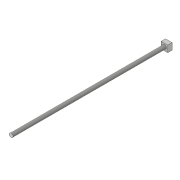
# Autodesk Inventor part: SA
Saved by Autodesk Inventor 2019 (Build 230136000, 136)
## iProperties
Created: 2019-10-07
Part Number: SA
Material: Generic
Document SubType Name: Modeling
Designer: Admin
Density: 1 g/cm^3
Appearance: Default
Author: Admin
Autodesk Inventor part; units mm, degrees
ref_plane "YZ Plane" through (0, 0, 0) normal (1, 0, 0) x (0, 1, 0)
ref_plane "XZ Plane" through (0, 0, 0) normal (0, 1, 0) x (-1, 0, 0)
ref_plane "XY Plane" through (0, 0, 0) normal (0, 0, 1) x (1, 0, 0)
sketch "Sketch1" plane through (0, 0, 0) normal (0, 0, 1) x (1, 0, 0)
  line L0 (0, 0) -> (15, 0)
  line L1 (15, 0) -> (15, 15)
  line L2 (15, 15) -> (0, 15)
  line L3 (0, 15) -> (0, 0)
  dimension "d0" = 15
  dimension "d1" = 15
  constraints: 8 end point, 2 parallel, 1 horizontal, 1 perpendicular
  measures "d0" distance of L2.end L1.end
  measures "d1" distance of L1.end L0.end
extrude "Extrusion1" add sketch "Sketch1" along normal blind 10
sketch "Sketch2" plane through (0, 0, 10) normal (0, 0, 1) x (1, 0, 0)
  line L0 (0, 15) -> (7.1003, 15)
  line L1 (15, 15) -> (0, 15) projected
  line L2 (7.5, 15) -> (7.5, 0)
  line L3 (0, 15) -> (7.9375, 15)
  line L4 (0, 0) -> (0, 7.9375)
  line L5 (0, 7.9375) -> (15, 7.9375)
  circle A0 centre (7.5, 7.9375) radius 4.5
  dimension "d15" = 9
  constraints: 10 end point, 2 midpoint, 2 point on line, 1 centre point, 1 perpendicular, 1 vertical
  measures "d15" diameter of A0
extrude "Extrusion2" add sketch "Sketch2" along normal blind 250
thread "Thread1" size "M11x1.5" class "6g" standard "ANSI Metric M Profile" full length
ref_plane "Work Plane1" through (7.5, 7.9375, 260) normal (0, 0, 1) x (1, 0, 0)
sketch "Sketch3" plane through (7.5, 7.9375, 260) normal (0, 0, 1) x (1, 0, 0)
  circle A0 centre (0, 0) radius 5.5 projected
  circle A1 centre (0, 0) radius 4.5
  point P0 (-7.5, -7.9375)
  dimension "d10" = 9
  constraints: 1 centre point, 1 coincident
  measures "d10" diameter of A1
extrude "Extrusion3" add sketch "Sketch3" along normal blind 100 contours A1
thread "Thread2" size "M9x1.25" class "6g" standard "ANSI Metric M Profile" full length
body "Solid1"
